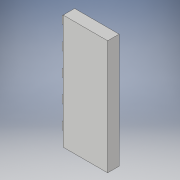
# Autodesk Inventor part: door (right side) 2nd map
Saved by Autodesk Inventor 2017 (Build 210142000, 142)
## iProperties
Created: 2018-05-21
Part Number: door (right side) 2nd map
Material: Generic
Document SubType Name: Modeling
Designer: braxtonwright
Density: 1 g/cm^3
Appearance: Default
Author: braxtonwright
Autodesk Inventor part; units mm, degrees
ref_plane "YZ Plane" through (0, 0, 0) normal (1, 0, 0) x (0, 1, 0)
ref_plane "XZ Plane" through (0, 0, 0) normal (0, 1, 0) x (-1, 0, 0)
ref_plane "XY Plane" through (0, 0, 0) normal (0, 0, 1) x (1, 0, 0)
sketch "Sketch1" plane through (0, 0, 0) normal (0, 0, 1) x (1, 0, 0)
  line L0 (0, 0) -> (88.9, 0)
  line L1 (88.9, 0) -> (88.9, 228.6)
  line L2 (88.9, 228.6) -> (0, 228.6)
  line L3 (0, 228.6) -> (0, 0)
  dimension "d0" = 88.9
  dimension "d1" = 228.6
  constraints: 8 end point, 2 parallel, 1 horizontal, 1 perpendicular
  measures "d0" distance of L2.end L1.end
  measures "d1" distance of L0.end L1.end
extrude "door" add sketch "Sketch1" along normal mid plane 22.86
sketch "Sketch2" plane through (0, 0, 0) normal (0, 0, 1) x (1, 0, 0)
  line L0 (88.9, 228.6) -> (0, 228.6) projected
  line L1 (88.9, 0) -> (0, 0) projected
  line L2 (4.4901, 64.0899) -> (4.4901, 50.2101)
  line L3 (4.4901, 50.2101) -> (0, 45.72)
  line L4 (0, 45.72) -> (-4.4901, 41.2299)
  line L5 (-4.4901, 41.2299) -> (-4.4901, 27.3501)
  line L6 (-4.4901, 27.3501) -> (0, 22.86)
  line L7 (0, 22.86) -> (0, 45.72)
  line L8 (0, 22.86) -> (4.4901, 18.3699)
  line L9 (4.4901, 18.3699) -> (4.4901, 4.4901)
  line L10 (4.4901, 4.4901) -> (0, 0)
  line L11 (0, 0) -> (0, 22.86)
  line L12 (0, 45.72) -> (0, 68.58)
  line L13 (-4.4901, 178.3899) -> (-4.4901, 164.5101)
  line L14 (0, 160.02) -> (0, 182.88)
  line L15 (-4.4901, 164.5101) -> (0, 160.02)
  line L16 (0, 160.02) -> (4.4901, 155.5299)
  line L17 (4.4901, 155.5299) -> (4.4901, 141.6501)
  line L18 (4.4901, 141.6501) -> (0, 137.16)
  line L19 (0, 137.16) -> (0, 160.02)
  line L20 (0, 137.16) -> (-4.4901, 132.6699)
  line L21 (-4.4901, 132.6699) -> (-4.4901, 118.7901)
  line L22 (0, 114.3) -> (0, 137.16)
  line L23 (-4.4901, 118.7901) -> (0, 114.3)
  line L24 (0, 114.3) -> (4.4901, 109.8099)
  line L25 (-4.4901, 73.0701) -> (0, 68.58)
  line L26 (-4.4901, 86.9499) -> (-4.4901, 73.0701)
  line L27 (0, 68.58) -> (0, 91.44)
  line L28 (0, 91.44) -> (-4.4901, 86.9499)
  line L29 (4.4901, 95.9301) -> (0, 91.44)
  line L30 (4.4901, 109.8099) -> (4.4901, 95.9301)
  line L31 (0, 91.44) -> (0, 114.3)
  line L32 (0, 68.58) -> (4.4901, 64.0899)
  line L33 (0, 228.6) -> (-4.4901, 224.1099)
  line L34 (0, 182.88) -> (-4.4901, 178.3899)
  line L35 (4.4901, 187.3701) -> (0, 182.88)
  line L36 (4.4901, 201.2499) -> (4.4901, 187.3701)
  line L37 (0, 182.88) -> (0, 205.74)
  line L38 (0, 205.74) -> (4.4901, 201.2499)
  line L39 (-4.4901, 210.2301) -> (0, 205.74)
  line L40 (-4.4901, 224.1099) -> (-4.4901, 210.2301)
  line L41 (0, 205.74) -> (0, 228.6)
  point P0 (-4.4901, 34.29)
  point P1 (4.4901, 57.15)
  point P2 (-4.4901, 80.01)
  point P3 (4.4901, 102.87)
  point P4 (-4.4901, 125.73)
  point P5 (4.4901, 148.59)
  point P6 (-4.4901, 171.45)
  point P7 (4.4901, 194.31)
  point P8 (-4.4901, 217.17)
  dimension "d36" = 6.35
  dimension "d37" = 228.6
  dimension "d38" = 11.43
  dimension "d39" = 11.43
  dimension "d40" = 11.43
  dimension "d41" = 11.43
  dimension "d42" = 11.43
  dimension "d43" = 11.43
  dimension "d44" = 11.43
  dimension "d45" = 11.43
  dimension "d46" = 45
  dimension "d47" = 45
  constraints: 80 end point, 14 point on line, 11 equal length, 9 collinear, 9 midpoint, 8 perpendicular, 6 vertical
  measures "d36" distance of L0.end L40.start
  measures "d37" distance of L1.end L0.end
  measures "d38" vertical distance of point (4.49, 194.31) L38.start
  measures "d39" vertical distance of L14.end point (-4.49, 171.45)
  measures "d40" vertical distance of L16.start point (4.49, 148.59)
  measures "d41" vertical distance of point (-4.49, 125.73) L19.start
  measures "d42" vertical distance of point (4.49, 102.87) L31.end
  measures "d43" vertical distance of point (-4.49, 80.01) L27.end
  measures "d44" vertical distance of point (4.49, 57.15) L12.end
  measures "d45" vertical distance of point (-4.49, 34.29) L12.start
  measures "d46" angle of L33 L41
  measures "d47" angle of L41 L39
extrude "teeth cut" cut sketch "Sketch2" along normal mid plane 17.78 contours L8 L9 L10 L11 | L37 L38 L36 L35 | L19 L16 L17 L18 | L31 L24 L30 L29 | L2 L3 L12 L32
extrude "teeth make" add sketch "Sketch2" along normal mid plane 17.78 contours L7 L6 L5 L4 | L39 L40 L33 L41 | L15 L13 L34 L14 | L23 L21 L20 L22 | L25 L26 L28 L27
equation "\"d38\" = d48"
equation "\"d39\" = d48"
equation "\"d40\" = d48"
equation "\"d41\" = d48"
equation "\"d42\" = d48"
equation "\"d43\" = d48"
equation "\"d44\" = d48"
equation "\"d45\" = d48"
equation "\"d21\" = d19"
equation "\"d48\" = 0.05 * d37"
equation "\"d19\" = 17.78"
body "Solid1"
